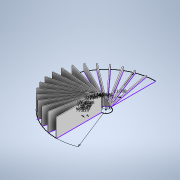
# Autodesk Inventor part: tiles
Saved by Autodesk Inventor 2020 (Build 240168000, 168)
## iProperties
Created: 2021-03-23
Part Number: tiles
Material: Generic
Document SubType Name: Modeling
Designer: tdmp4
Density: 1 g/cm^3
Appearance: Default
Author: tdmp4
Autodesk Inventor part; units mm, degrees
ref_plane "YZ Plane" through (0, 0, 0) normal (1, 0, 0) x (0, 1, 0)
ref_plane "XZ Plane" through (0, 0, 0) normal (0, 1, 0) x (-1, 0, 0)
ref_plane "XY Plane" through (0, 0, 0) normal (0, 0, 1) x (1, 0, 0)
sketch "Sketch8" plane through (0, 0, 0) normal (0, 1, 0) x (-1, 0, 0)
  circle A0 centre (0, 0) radius 12.7
  arc A1 (0, -139.7) -> (0, 139.7) centre (0, 0) ccw
  line L0 (0, -12.7) -> (0, -139.7)
  line L1 (0, 12.7) -> (0, 139.7)
  line L2 (2.3336, -12.4838) -> (25.6698, -137.3213)
  line L3 (0, 0) -> (139.7, 0) construction
  line L4 (4.5878, -11.8424) -> (50.4655, -130.2664)
  line L5 (0, 0) -> (139.7, 0) construction
  line L6 (6.6857, -10.7978) -> (73.5426, -118.7753)
  line L7 (0, 0) -> (139.7, 0) construction
  line L8 (8.5559, -9.3854) -> (94.1153, -103.2395)
  line L9 (0, 0) -> (139.7, 0) construction
  line L10 (10.1348, -7.6535) -> (111.483, -84.1881)
  line L11 (0, 0) -> (139.7, 0) construction
  line L12 (11.3686, -5.6609) -> (125.0543, -62.2696)
  line L13 (0, 0) -> (139.7, 0) construction
  line L14 (12.2152, -3.4755) -> (134.367, -38.2307)
  line L15 (0, 0) -> (139.7, 0) construction
  line L16 (12.6458, -1.1718) -> (139.1041, -12.8899)
  line L17 (0, 0) -> (139.7, 0) construction
  line L18 (12.6458, 1.1718) -> (139.1041, 12.8899)
  line L19 (0, 0) -> (139.7, 0) construction
  line L20 (12.2152, 3.4755) -> (134.367, 38.2307)
  line L21 (0, 0) -> (139.7, 0) construction
  line L22 (0, 0) -> (139.7, 0) construction
  line L23 (11.3686, 5.6609) -> (125.0543, 62.2696)
  line L24 (0, 0) -> (139.7, 0) construction
  line L25 (10.1348, 7.6535) -> (111.483, 84.1881)
  line L26 (0, 0) -> (139.7, 0) construction
  line L27 (8.5559, 9.3854) -> (94.1153, 103.2395)
  line L28 (0, 0) -> (139.7, 0) construction
  line L29 (6.6857, 10.7978) -> (73.5426, 118.7753)
  line L30 (0, 0) -> (139.7, 0) construction
  line L31 (6.6857, 10.7978) -> (74.8165, 120.8327)
  line L32 (0, 0) -> (142.1199, 0) construction
  line L33 (4.5878, 11.8424) -> (50.4655, 130.2664)
  line L34 (0, 0) -> (139.7, 0) construction
  line L35 (2.3336, 12.4838) -> (25.6698, 137.3213)
  line L36 (0, 0) -> (139.7, 0) construction
  line L37 (2.3336, -12.4838) -> (0, -12.7)
  line L38 (2.3336, -12.4838) -> (4.5878, -11.8424)
  line L39 (4.5878, -11.8424) -> (6.6857, -10.7978)
  line L40 (6.6857, -10.7978) -> (8.5559, -9.3854)
  line L41 (8.5559, -9.3854) -> (10.1348, -7.6535)
  line L42 (10.1348, -7.6535) -> (11.3686, -5.6609)
  line L43 (11.3686, -5.6609) -> (12.2152, -3.4755)
  line L44 (12.2152, -3.4755) -> (12.6458, -1.1718)
  line L45 (12.6458, -1.1718) -> (12.6458, 1.1718)
  line L46 (12.6458, 1.1718) -> (12.2152, 3.4755)
  line L47 (12.2152, 3.4755) -> (11.3686, 5.6609)
  line L48 (11.3686, 5.6609) -> (10.1348, 7.6535)
  line L49 (10.1348, 7.6535) -> (8.5559, 9.3854)
  line L50 (8.5559, 9.3854) -> (6.6857, 10.7978)
  line L51 (6.6857, 10.7978) -> (4.5878, 11.8424)
  line L52 (4.5878, 11.8424) -> (2.3336, 12.4838)
  line L53 (2.3336, 12.4838) -> (0, 12.7)
  line L54 (0, -12.7) -> (23.3723, -137.731)
  line L55 (0, -12.7) -> (127.1967, -12.7) construction
  line L56 (2.3336, -12.4838) -> (48.2824, -131.0912)
  line L57 (2.3336, -12.4838) -> (129.5304, -12.4838) construction
  line L58 (4.5878, -11.8424) -> (71.0599, -120.2771)
  line L59 (6.6857, -10.7978) -> (92.3776, -104.7973)
  line L60 (8.5559, -9.3854) -> (110.0938, -86.0632)
  line L61 (8.5559, -9.3854) -> (135.7936, -9.3854) construction
  line L62 (10.1348, -7.6535) -> (123.9967, -64.3499)
  line L63 (10.1348, -7.6535) -> (137.3316, -7.6535) construction
  line L64 (11.3686, -5.6609) -> (133.7097, -40.4699)
  line L65 (11.3686, -5.6609) -> (138.5653, -5.6609) construction
  line L66 (12.2152, -3.4755) -> (138.8693, -15.2118)
  line L67 (12.2152, -3.4755) -> (139.4119, -3.4755) construction
  line L68 (12.6458, -1.1718) -> (139.3, 10.5644)
  line L69 (12.6458, 1.1718) -> (134.9869, 35.9809)
  line L70 (11.3686, 5.6609) -> (125.0543, 62.2696)
  line L71 (11.3686, 5.6609) -> (138.3686, 5.6609) construction
  line L72 (12.2152, 3.4755) -> (126.1445, 60.0305)
  line L73 (12.2152, 3.4755) -> (139.4093, 3.4755) construction
  line L74 (11.3686, 5.6609) -> (112.8738, 82.314)
  line L75 (11.3686, 5.6609) -> (138.5653, 5.6609) construction
  line L76 (10.1348, 7.6535) -> (95.8267, 101.653)
  line L77 (10.1348, 7.6535) -> (137.3316, 7.6535) construction
  line L78 (8.5559, 9.3854) -> (75.5164, 117.5303)
  line L79 (6.6857, 10.7978) -> (52.6345, 129.4052)
  line L80 (6.6857, 10.7978) -> (133.8824, 10.7978) construction
  line L81 (4.5878, 11.8424) -> (27.9601, 136.8734)
  line L82 (4.5878, 11.8424) -> (131.7845, 11.8424) construction
  line L83 (2.3336, 12.4838) -> (2.3336, 139.6805)
  point P0 (110.0611, -86.0386)
  dimension "d20" = 25.4
  dimension "d21" = 279.4
  dimension "d22" = 79.412
  dimension "d23" = 68.823
  dimension "d24" = 58.235
  dimension "d25" = 47.647
  dimension "d26" = 37.059
  dimension "d27" = 26.471
  dimension "d28" = 15.882
  dimension "d29" = 5.294
  dimension "d30" = 5.294
  dimension "d31" = 15.882
  dimension "d33" = 26.471
  dimension "d34" = 37.059
  dimension "d35" = 47.647
  dimension "d36" = 58.235
  dimension "d37" = 58.235
  dimension "d38" = 68.823
  dimension "d39" = 79.412
  dimension "d40" = 79.412
  dimension "d41" = 68.823
  dimension "d42" = 37.059
  dimension "d43" = 26.471
  dimension "d44" = 15.882
  dimension "d45" = 5.294
  dimension "d46" = 26.471
  dimension "d47" = 26.4
  dimension "d48" = 37.059
  dimension "d49" = 47.647
  dimension "d50" = 68.823
  dimension "d51" = 79.412
  constraints: 168 end point, 30 horizontal, 12 equal length, 4 parallel, 3 vertical, 2 coincident, 1 collinear, 56 other
  measures "d22" angle of L2 L3
  measures "d23" angle of L4 L5
  measures "d24" angle of L6 L7
  measures "d25" angle of L8 L9
  measures "d26" angle of L10 L11
  measures "d27" angle of L12 L13
  measures "d28" angle of L14 L15
  measures "d29" angle of L16 L17
  measures "d30" angle of L19 L18
  measures "d31" angle of L21 L20
  measures "d33" angle of L24 L23
  measures "d34" angle of L26 L25
  measures "d35" angle of L28 L27
  measures "d36" angle of L30 L29
  measures "d37" angle of L32 L31
  measures "d38" angle of L34 L33
  measures "d39" angle of L36 L35
  measures "d40" angle of L54 L55
  measures "d41" angle of L56 L57
  measures "d42" angle of L60 L61
  measures "d43" angle of L62 L63
  measures "d44" angle of L64 L65
  measures "d45" angle of L66 L67
  measures "d46" angle of L71 L70
  measures "d47" angle of L73 L72
  measures "d48" angle of L75 L74
  measures "d49" angle of L77 L76
  measures "d50" angle of L80 L79
  measures "d51" angle of L82 L81
extrude "Extrusion6" add sketch "Sketch8" along normal blind 3.175 contours L2 A1 L54 A0
extrude "Extrusion7" add sketch "Sketch8" along normal blind 6.35 contours L4 A1 L56 A0
extrude "Extrusion8" add sketch "Sketch8" along normal blind 9.525 contours L6 A1 L58 A0
extrude "Extrusion9" add sketch "Sketch8" along normal blind 12.7 contours L8 A1 L59 A0
extrude "Extrusion10" add sketch "Sketch8" along normal blind 15.875 contours L10 A1 L60 A0
extrude "Extrusion11" add sketch "Sketch8" along normal blind 19.05 contours L12 A1 L62 A0
extrude "Extrusion12" add sketch "Sketch8" along normal blind 22.225 contours L14 A1 L64 A0
extrude "Extrusion13" add sketch "Sketch8" along normal blind 25.4 contours L16 A1 L66 A0
extrude "Extrusion14" add sketch "Sketch8" along normal blind 28.575 contours A0 L18 A1 L68
extrude "Extrusion15" add sketch "Sketch8" along normal blind 31.75 contours A0 L20 A1 L69
extrude "Extrusion16" add sketch "Sketch8" along normal blind 34.925 contours A0 L23 A1 L72
extrude "Extrusion17" add sketch "Sketch8" along normal blind 38.1 contours A0 L25 A1 L74
extrude "Extrusion18" add sketch "Sketch8" along normal blind 41.275 contours A0 L27 A1 L76
extrude "Extrusion19" add sketch "Sketch8" along normal blind 44.45 contours A0 L29 A1 L78
extrude "Extrusion20" add sketch "Sketch8" along normal blind 47.625 contours A0 L33 A1 L79
extrude "Extrusion21" add sketch "Sketch8" along normal blind 50.8 contours A0 L35 A1 L81
extrude "Extrusion22" add sketch "Sketch8" along normal blind 50.8 contours A0 L1 A1 L83
body "Solid2"
